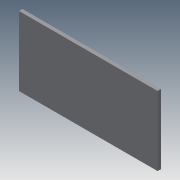
# Autodesk Inventor part: baseboard
Saved by Autodesk Inventor 2015 (Build 190159000, 159)
## iProperties
Created: 2014-07-22
Part Number: baseboard
Material: Generic
Document SubType Name: Modeling
Designer: shohei
Density: 1 g/cm^3
Appearance: Default
Mass: 400 g
Surface Area: 900 cm^2
Volume: 400 cm^3
Author: shohei
Autodesk Inventor part; units mm, degrees
ref_plane "YZ Plane" through (0, 0, 0) normal (1, 0, 0) x (0, 1, 0)
ref_plane "XZ Plane" through (0, 0, 0) normal (0, 1, 0) x (-1, 0, 0)
ref_plane "XY Plane" through (0, 0, 0) normal (0, 0, 1) x (1, 0, 0)
sketch "Sketch1" plane through (0, 0, 0) normal (0, 1, 0) x (-1, 0, 0)
  line L0 (-200, -100) -> (200, -100)
  line L1 (200, -100) -> (200, 100)
  line L2 (200, 100) -> (-200, 100)
  line L3 (-200, 100) -> (-200, -100)
  line L4 (-200, -100) -> (200, 100) construction
  line L5 (200, -100) -> (-200, 100) construction
  point P0 (0, 0)
  dimension "d0" = 400
  dimension "d1" = 200
  constraints: 12 end point, 2 midpoint, 2 parallel, 1 horizontal, 1 perpendicular
  measures "d0" distance of L2.end L1.end
  measures "d1" distance of L1.end L0.end
extrude "Extrusion1" add sketch "Sketch1" along normal blind 10
body "Solid1"
